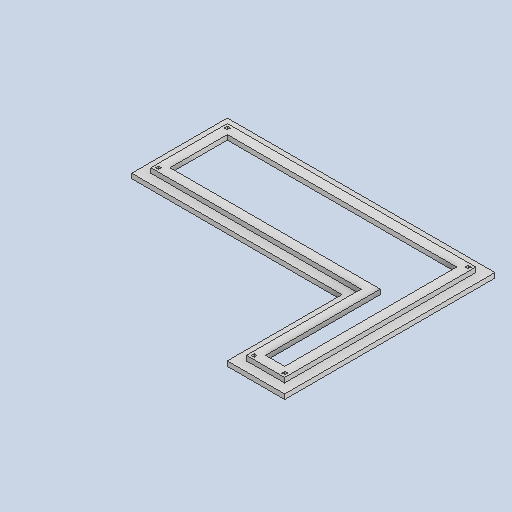
# Autodesk Inventor part: base down
Saved by Autodesk Inventor 2025.3 (Build 293356000, 356)
## iProperties
Created: 2026-05-24
Part Number: base down
Material: Generic
Document SubType Name: Modeling
Designer: kamal
Density: 1 g/cm^3
Appearance: Default
Author: kamal
Autodesk Inventor part; units mm, degrees
ref_plane "YZ Plane" through (0, 0, 0) normal (1, 0, 0) x (0, 1, 0)
ref_plane "XZ Plane" through (0, 0, 0) normal (0, 1, 0) x (-1, 0, 0)
ref_plane "XY Plane" through (0, 0, 0) normal (0, 0, 1) x (1, 0, 0)
sketch "Sketch1" plane through (0, 0, 0) normal (0, 1, 0) x (-1, 0, 0)
  line L0 (0, 0) -> (80, 0)
  line L1 (80, 0) -> (80, -240)
  line L2 (80, -400) -> (0, -400)
  line L3 (0, -400) -> (0, 0)
  line L4 (80, -400) -> (520, -400)
  line L5 (520, -400) -> (520, -240)
  line L6 (520, -240) -> (80, -240)
  line L7 (540, -420) -> (80, -420)
  line L8 (80, -420) -> (-20, -420)
  line L9 (-20, -420) -> (-20, 20)
  line L10 (-20, 20) -> (100, 20)
  line L11 (100, 20) -> (100, -220)
  line L12 (100, -220) -> (540, -220)
  line L13 (540, -220) -> (540, -420)
  line L14 (500, -380) -> (80, -380)
  line L15 (80, -380) -> (20, -380)
  line L16 (20, -380) -> (20, -20)
  line L17 (20, -20) -> (60, -20)
  line L18 (60, -20) -> (60, -260)
  line L19 (60, -260) -> (500, -260)
  line L20 (500, -260) -> (500, -380)
  dimension "d5" = 400
  dimension "d6" = 160
  dimension "d7" = 80
  dimension "d8" = 440
  dimension "d9" = 20
  dimension "d10" = 20
  constraints: 42 end point, 9 parallel, 6 perpendicular, 2 horizontal, 1 vertical, 12 other
  measures "d5" distance of L2.end L0.start
  measures "d6" distance of L4.end L5.end
  measures "d7" distance of L0.start L0.end
  measures "d8" distance from line of L2.start L5
  measures "d9" distance between parallel lines of L4 L7
  measures "d10" distance between parallel lines of L4 L14
extrude "Extrusion2" add sketch "Sketch1" against normal blind 10 contours L7 L8 L9 L10 L11 L12 L13
extrude "Extrusion3" add sketch "Sketch1" along normal blind 10 contours L0 L1 L6 L5 L4 L2 L3
sketch "Sketch2" plane through (0, 10, 0) normal (0, 1, 0) x (1, 0, 0)
  line L0 (-11, 11) -> (-5, 11)
  line L1 (-5, 11) -> (-5, 5)
  line L2 (-5, 5) -> (-11, 5)
  line L3 (-11, 5) -> (-11, 11)
  line L4 (-520, 400) -> (-520, 240) projected
  line L5 (-520, 240) -> (-80, 240) projected
  line L6 (-80, 240) -> (-80, 0) projected
  line L7 (-80, 0) -> (0, 0) projected
  line L8 (0, 0) -> (0, 400) projected
  line L9 (0, 400) -> (-520, 400) projected
  line L10 (-500, 380) -> (-20, 380) projected
  line L11 (-20, 380) -> (-20, 20) projected
  line L12 (-20, 20) -> (-60, 20) projected
  line L13 (-60, 20) -> (-60, 260) projected
  line L14 (-60, 260) -> (-500, 260) projected
  line L15 (-500, 260) -> (-500, 380) projected
  line L16 (-40, 0) -> (-40, 400)
  line L17 (-69, 11) -> (-75, 11)
  line L18 (-75, 11) -> (-75, 5)
  line L19 (-75, 5) -> (-69, 5)
  line L20 (-69, 5) -> (-69, 11)
  line L21 (-40, 200) -> (0, 200)
  line L22 (-11, 389) -> (-5, 389)
  line L23 (-5, 389) -> (-5, 395)
  line L24 (-5, 395) -> (-11, 395)
  line L25 (-11, 395) -> (-11, 389)
  line L26 (-500, 320) -> (-40, 320)
  line L27 (-509, 389) -> (-515, 389)
  line L28 (-515, 389) -> (-515, 395)
  line L29 (-515, 395) -> (-509, 395)
  line L30 (-509, 395) -> (-509, 389)
  line L31 (-509, 251) -> (-515, 251)
  line L32 (-515, 251) -> (-515, 245)
  line L33 (-515, 245) -> (-509, 245)
  line L34 (-509, 245) -> (-509, 251)
  dimension "d19" = 6
  dimension "d20" = 6
  dimension "d21" = 5
  dimension "d22" = 11
  dimension "d23" = 6
  dimension "d24" = 11
  dimension "d25" = 11
  constraints: 46 end point, 12 symmetric about line, 5 perpendicular, 4 midpoint, 4 parallel, 2 horizontal, 2 point on line
  measures "d19" distance of L1.end L2.end
  measures "d20" distance of L0.end L1.end
  measures "d21" distance from line of point (0, 0) L1
  measures "d22" distance from line of point (0, 0) L0
  measures "d23" distance of L27.end L28.end
  measures "d24" distance between parallel lines of L4 L30
  measures "d25" distance between parallel lines of L9 L27
extrude "Extrusion4" cut sketch "Sketch2" against normal through all contours L0 L1 L2 L3 | L20 L19 L18 L17 | L25 L24 L23 L22 | L27 L28 L29 L30 | L34 L33 L32 L31
body "Solid2"
